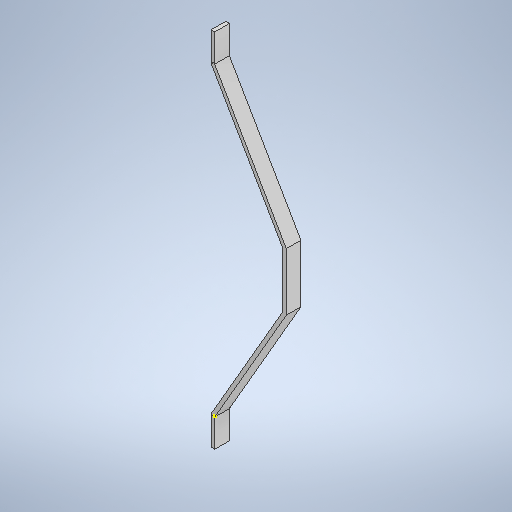
# Autodesk Inventor part: AçoChato
Saved by Autodesk Inventor 2025 (Build 290162010, 162A)
## iProperties
Created: 2024-11-28
Part Number: AçoChato
Material: Generic
Document SubType Name: Modeling
Designer: Bryan Ss
Density: 1 g/cm^3
Appearance: Default
Author: Bryan Ss
Autodesk Inventor part; units mm, degrees
ref_plane "YZ Plane" through (0, 0, 0) normal (1, 0, 0) x (0, 1, 0)
sketch "Sketch1" plane through (0, 0, 0) normal (0, 1, 0) x (-1, 0, 0)
  line L0 (0, 0) -> (6.35, 0)
  line L1 (6.35, 0) -> (6.35, -25.4)
  line L2 (6.35, -25.4) -> (0, -25.4)
  line L3 (0, -25.4) -> (0, 0)
  dimension "d0" = 6.35
  dimension "d1" = 25.4
  constraints: 8 end point, 2 parallel, 1 horizontal, 1 perpendicular
  measures "d0" distance of L1.end L2.end
  measures "d1" distance of L0.end L1.end
extrude "Extrusion1" add sketch "Sketch1" along normal blind 50
sketch "Sketch2" plane through (0, 50, 0) normal (0, 1, 0) x (1, 0, 0)
  point P0 (0, 0)
ref_plane "Work Plane2" through (-6.35, 50, -25.4) normal (0.5, 0.866, 0) x (0, 0, 1)
sketch "Sketch3" plane through (-6.35, 50, -25.4) normal (0.5, 0.866, 0) x (0, 0, 1)
  line L0 (25.5214, 0) -> (0.1214, 0)
  line L1 (0.1214, 0) -> (0.1214, 6.35)
  line L2 (0.1214, 6.35) -> (25.5214, 6.35)
  line L3 (25.5214, 6.35) -> (25.5214, 0)
  point P0 (25.4, 30.4993)
  dimension "d5" = 25.4
  dimension "d6" = 6.35
  constraints: 8 end point, 2 parallel, 1 horizontal, 1 perpendicular
  measures "d5" distance of L1.end L2.end
  measures "d6" distance of L0.end L1.end
extrude "Extrusion2" add sketch "Sketch3" along normal blind 250
ref_plane "Work Plane3" through (124.1493, 263.3314, 0.1214) normal (0, 1, 0) x (0, 0, -1)
sketch "Sketch4" plane through (124.1493, 263.3314, 0.1214) normal (0, 1, 0) x (0, 0, -1)
  line L0 (25.4, 124.1493) -> (25.4, 0) projected
  line L1 (25.4, 0) -> (0, 0)
  line L2 (0, 0) -> (0, 6.35)
  line L3 (0, 6.35) -> (25.4, 6.35)
  line L4 (25.4, 6.35) -> (25.4, 0)
  point P0 (0.1214, 124.1493)
  point P1 (25.4, 6.35)
  dimension "d10" = 25.4
  dimension "d11" = 6.35
  constraints: 8 end point, 2 parallel, 1 horizontal, 1 perpendicular
  measures "d10" distance of L2.end L3.end
  measures "d11" distance of L1.end L2.end
extrude "Extrusion3" add sketch "Sketch4" along normal blind 50
mirror "Mirror1" about plane through (120.9743, 313.3314, -12.5786) normal (0, 1, 0) of "Extrusion1", "Extrusion2", "Extrusion3"
body "Solid1"
